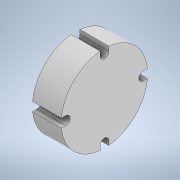
# Autodesk Inventor part: 711114
Saved by Autodesk Inventor 2022 (Build 260153000, 153)
## iProperties
Created: 2021-10-21
Part Number: 711114
Material: Типовые
Document SubType Name: Modeling
Designer: RaNSiD
Density: 1 g/cm^3
Appearance: По умолчанию
Author: RaNSiD
Autodesk Inventor part; units mm, degrees
ref_plane "YZ Plane" through (0, 0, 0) normal (1, 0, 0) x (0, 1, 0)
ref_plane "XZ Plane" through (0, 0, 0) normal (0, 1, 0) x (-1, 0, 0)
ref_plane "XY Plane" through (0, 0, 0) normal (0, 0, 1) x (1, 0, 0)
sketch "Эскиз1" plane through (0, 0, 0) normal (0, 0, 1) x (1, 0, 0)
  line L0 (0, 0) -> (20, 0)
  line L1 (20, 0) -> (20, 30)
  line L2 (20, 30) -> (0, 30)
  line L3 (0, 30) -> (0, 0)
  dimension "d0" = 20
  dimension "d1" = 30
  constraints: 8 end point, 2 parallel, 1 horizontal, 1 perpendicular
  measures "d0" distance of L2.end L1.end
  measures "d1" distance of L1.end L0.end
revolve "Вращение1" add sketch "Эскиз1" angle 360 about axis through (0, 0, 0) along (1, 0, 0)
sketch "Эскиз2" plane through (0, 0, 0) normal (-1, 0, 0) x (0, 0, 1)
  circle A0 centre (0, 0) radius 30 construction
  circle A1 centre (0, 0) radius 30 projected
  line L0 (-3, 29.8496) -> (-3, 26.8496)
  line L1 (3, 29.8496) -> (3, 26.8496)
  arc A2 (-3, 26.8496) -> (3, 26.8496) centre (0, 26.8496) ccw
  line L2 (-29.8496, -3) -> (-26.8496, -3)
  line L3 (-29.8496, 3) -> (-26.8496, 3)
  arc A3 (-26.8496, -3) -> (-26.8496, 3) centre (-26.8496, 0) ccw
  line L4 (3, -29.8496) -> (3, -26.8496)
  line L5 (-3, -29.8496) -> (-3, -26.8496)
  arc A4 (3, -26.8496) -> (-3, -26.8496) centre (0, -26.8496) ccw
  line L6 (29.8496, 3) -> (26.8496, 3)
  line L7 (29.8496, -3) -> (26.8496, -3)
  arc A5 (26.8496, 3) -> (26.8496, -3) centre (26.8496, 0) ccw
  dimension "d3" = 3
  dimension "d4" = 3
  dimension "d5" = 3
  dimension "d8" = 360
  constraints: 16 end point, 10 point on circle, 4 centre point, 2 horizontal alignment, 2 vertical, 1 coincident, 1 tangent, 33 other
  measures "d3" distance of L0.start L0.end
  measures "d4" distance of L1.start L1.end
  measures "d5" radius of A2
extrude "Выдавливание1" cut sketch "Эскиз2" against normal blind 20 contours A1 L7 A5 L6 | L1 A2 L0 A1 | A1 L5 A4 L4 | L3 A3 L2 A1
sketch "Эскиз3" plane through (0, 0, 26.8496) normal (-1, 0, 0) x (0, 0, 1)
  line L0 (-26.8496, 0) -> (-21.8496, 0) construction
  dimension "d12" = 5
  constraints: 2 end point, 1 coincident, 1 horizontal
  measures "d12" distance of L0.start L0.end
hole "Отверстие1" at (0, 0, 5) direction (1, 0, 0) diameter 14 depth 8 tip angle 118 countersink diameter 19 countersink angle 90
